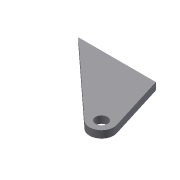
# Autodesk Inventor part: Soporte resorte freno
Saved by Autodesk Inventor 2019 (Build 230136000, 136)
## iProperties
Created: 2020-02-07
Part Number: Soporte resorte freno
Material: Generic
Document SubType Name: Modeling
Designer: Juan Carlos Botero
Density: 1 g/cm^3
Appearance: Default
Author: Juan Carlos Botero
Autodesk Inventor part; units mm, degrees
ref_plane "YZ Plane" through (0, 0, 0) normal (1, 0, 0) x (0, 1, 0)
ref_plane "XZ Plane" through (0, 0, 0) normal (0, 1, 0) x (-1, 0, 0)
ref_plane "XY Plane" through (0, 0, 0) normal (0, 0, 1) x (1, 0, 0)
sketch "Sketch1" plane through (0, 0, 0) normal (0, 1, 0) x (-1, 0, 0)
  circle A0 centre (0, 50) radius 5
  circle A1 centre (0, 50) radius 10
  line L0 (-9.5533, 47.0447) -> (5, 0)
  line L1 (5, 0) -> (69.1187, 0)
  line L2 (69.1187, 6) -> (69.1187, 0) projected
  line L3 (69.1187, 6) -> (6.3595, 57.7173)
  point P0 (0, 0)
  dimension "d0" = 10
  dimension "d1" = 50
  dimension "d2" = 20
  constraints: 6 end point, 2 centre point, 2 point on circle, 2 tangent, 1 coincident, 1 horizontal, 1 point on line, 1 vertical alignment
  measures "d0" diameter of A0
  measures "d1" distance of point (0, 0) A0.centre
  measures "d2" diameter of A1
extrude "Extrusion1" add sketch "Sketch1" along normal mid plane 6
body "Solid1"
